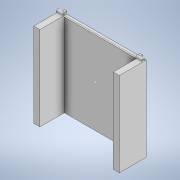
# Autodesk Inventor part: McCrea_body_zadok_walle
Saved by Autodesk Inventor 2022 (Build 260153000, 153)
## iProperties
Created: 2022-01-04
Part Number: McCrea_body_zadok_walle
Material: Generic
Document SubType Name: Modeling
Designer: Lukas
Density: 1 g/cm^3
Appearance: Default
Author: Lukas
Autodesk Inventor part; units mm, degrees
ref_plane "YZ Plane" through (0, 0, 0) normal (1, 0, 0) x (0, 1, 0)
ref_plane "XZ Plane" through (0, 0, 0) normal (0, 1, 0) x (-1, 0, 0)
ref_plane "XY Plane" through (0, 0, 0) normal (0, 0, 1) x (1, 0, 0)
sketch "Sketch1" plane through (0, 0, 0) normal (0, 0, 1) x (1, 0, 0)
  line L0 (39.6273, 34.4888) -> (39.6273, -34.5112)
  line L1 (39.6273, -34.5112) -> (-30.3727, -34.5112)
  line L2 (-30.3727, -34.5112) -> (-30.3727, 34.4888)
  line L3 (-27.3727, 34.4888) -> (36.6273, 34.4888)
  line L4 (36.6273, 34.4888) -> (36.6273, 36.4888)
  line L5 (36.6273, 36.4888) -> (-27.3727, 36.4888)
  line L6 (-27.3727, 36.4888) -> (-27.3727, 34.4888)
  line L7 (-27.3727, 34.4888) -> (-30.3727, 34.4888)
  line L8 (36.6273, 34.4888) -> (39.6273, 34.4888)
  point P0 (0, 0)
  dimension "d0" = 70
  dimension "d1" = 69
  dimension "d2" = 3
  dimension "d4" = 64
  dimension "d5" = 2
  constraints: 18 end point, 3 parallel, 2 horizontal, 2 perpendicular
  measures "d0" distance of L0.end L1.end
  measures "d1" distance of L0.start L0.end
  measures "d2" distance of L2.end L3.start
  measures "d4" distance of L5.end L4.end
  measures "d5" distance of L4.end L3.end
extrude "Extrusion1" add sketch "Sketch1" along normal blind 2
sketch "Sketch4" plane through (0, 0, 2) normal (0, 0, 1) x (1, 0, 0)
  point P0 (0, 0)
sketch "Sketch5" plane through (-27.3727, 34.4888, 0) normal (-1, 0, 0) x (0, 0, 1)
  line L0 (0, 0) -> (0, 2) projected
  line L1 (0, 1) -> (2.475, 1)
  circle A0 centre (2.475, 1) radius 1.214
  circle A1 centre (2.475, 1) radius 0.5
  point P0 (0, -34.4888)
  dimension "d14" = 2.475
  dimension "d15" = 2.428
  dimension "d16" = 1
  constraints: 2 centre point, 2 coincident, 2 end point, 1 horizontal, 1 midpoint
  measures "d14" distance of L1.start L1.end
  measures "d15" diameter of A0
  measures "d16" diameter of A1
extrude "Extrusion3" add sketch "Sketch5" along normal blind 3 and the other way blind 67
sketch "Sketch6" plane through (0, 0, 2) normal (0, 0, 1) x (1, 0, 0)
  line L0 (-27.3727, 34.4888) -> (-30.3727, 34.4888) projected
  line L1 (-30.3727, 34.4888) -> (-25.3727, 34.4888)
  line L2 (39.6273, -34.5112) -> (39.6273, 34.4888) projected
  line L3 (39.6273, 34.4888) -> (34.6273, 34.4888)
  line L4 (39.6273, 34.4888) -> (36.6273, 34.4888) projected
  line L5 (-25.3727, 34.4888) -> (34.6273, 34.4888)
  line L6 (34.6273, 34.4888) -> (34.6273, 37.3895)
  line L7 (34.6273, 37.3895) -> (-25.3727, 37.3895)
  line L8 (-25.3727, 37.3895) -> (-25.3727, 34.4888)
  point P0 (0, 0)
  dimension "d21" = 5
  dimension "d22" = 5
  constraints: 12 end point, 2 collinear, 2 parallel, 1 horizontal, 1 perpendicular
  measures "d21" distance of L0.end L1.end
  measures "d22" distance of L2.end L3.end
extrude "Extrusion4" cut sketch "Sketch6" along normal mid plane 5
sketch "Sketch7" plane through (0, 0, 2) normal (0, 0, 1) x (1, 0, 0)
  line L0 (-30.3727, 34.4888) -> (-30.3727, -34.5112) projected
  line L1 (-30.3727, -34.5112) -> (39.6273, -34.5112) projected
  line L2 (-30.3727, 34.4888) -> (-25.3727, 34.4888)
  line L3 (-25.3727, 34.4888) -> (-25.3727, -34.5112)
  line L4 (-25.3727, -34.5112) -> (-30.3727, -34.5112)
  line L5 (-30.3727, -34.5112) -> (-30.3727, 34.4888)
  line L6 (39.6273, 34.3716) -> (-30.3727, 34.3716) projected
  line L7 (39.6273, 34.3716) -> (34.6273, 34.3716)
  line L8 (34.6273, 34.3716) -> (34.6273, -34.5112)
  line L9 (34.6273, -34.5112) -> (39.6273, -34.5112)
  line L10 (39.6273, -34.5112) -> (39.6273, 34.3716)
  point P0 (0, 0)
  point P1 (39.6273, -34.5112)
  point P2 (-25.3727, 34.3716)
  dimension "d25" = 5
  dimension "d26" = 5
  constraints: 16 end point, 4 parallel, 2 horizontal, 2 perpendicular, 2 point on line
  measures "d25" distance of L3.end L4.end
  measures "d26" distance of L9.end L8.end
extrude "Extrusion5" add sketch "Sketch7" along normal blind 20 contours L6 L3 L1 L0 | L6 L10 L1 L8
sketch "Sketch8" plane through (-30.3727, -34.5112, 0) normal (-1, 0, 0) x (0, 0, 1)
  point P0 (0, 34.5112)
body "Solid1"
